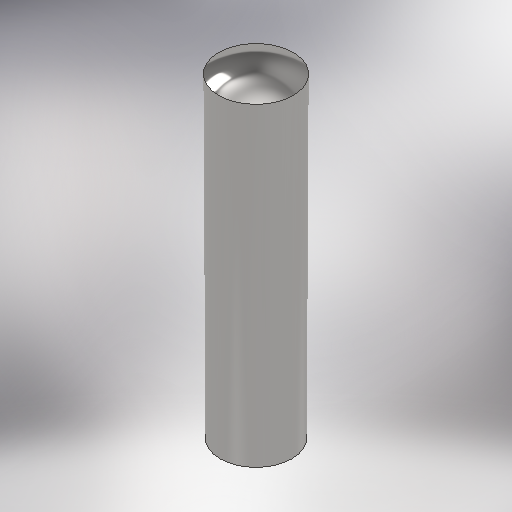
# Autodesk Inventor part: 定位销
Saved by Autodesk Inventor 2025 (Build 290162000, 162)
## iProperties
Created: 2025-03-16
Part Number: 定位销
Material: 常规
Document SubType Name: Modeling
Designer: ASUS
Density: 1 g/cm^3
Appearance: 钢 - 抛光
Author: ASUS
Autodesk Inventor part; units mm, degrees
ref_plane "YZ Plane" through (0, 0, 0) normal (1, 0, 0) x (0, 1, 0)
ref_plane "XY Plane" through (0, 0, 0) normal (0, 0, 1) x (1, 0, 0)
sketch "草图1" plane through (0, 0, 0) normal (1, 0, 0) x (0, 1, 0)
  line L0 (33.3814, 0) -> (-27.6379, 0)
  arc A0 (18.2824, 0) -> (17.2824, 4.0162) centre (9.7176, 0) ccw
  arc A1 (-16.7176, 3.873) -> (-17.7176, 0) centre (-9.7176, 0) ccw
  line L1 (17.2824, 4.0162) -> (-16.7176, 3.873)
  line L2 (0, -0.8155) -> (0, 4.893) projected
  point P0 (0, 0)
  dimension "d0" = 8.5648
  dimension "d1" = 8
  dimension "d2" = 1
  dimension "d3" = 1
  dimension "d4" = 36
  dimension "d6" = 89.759
  dimension "d9" = 18.2824
  dimension "d10" = 17.7176
  constraints: 5 point on line, 4 end point, 4 point on circle, 2 centre point, 1 horizontal, 1 symmetric about line
  measures "d0" radius of A0
  measures "d1" radius of A1
  measures "d2" horizontal distance of A0.start L1.start
  measures "d3" horizontal distance of A1.end L1.end
  measures "d4" distance of A1.end A0.start
  measures "d6" angle of L2 L1
  measures "d9" distance from line of L2 A0.start
  measures "d10" distance from line of L2 A1.end
revolve "旋转1" add sketch "草图1" angle 360 about axis through (0, 33.3814, 0) along (0, -1, 0)
ref_plane "工作平面1" through (0, 11.2824, 0) normal (0, 1, 0) x (-1, 0, 0)
ref_plane "工作平面2" through (0, -10.7176, 0) normal (0, 1, 0) x (-1, 0, 0)
equation "\"d0\" = r2"
equation "\"d1\" = r1"
equation "\"d2\" = a"
equation "\"d3\" = a"
equation "\"d4\" = l_"
equation "\"d\" = 8"
equation "\"a\" = 1"
equation "\"r1\" = d"
equation "\"l_\" = 36"
equation "\"r2\" = 8.5648"
